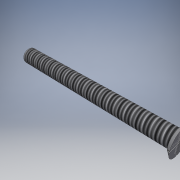
# Autodesk Inventor part: screws (for assembly)
Saved by Autodesk Inventor 2016 (Build 200138000, 138)
## iProperties
Created: 2017-10-23
Part Number: screws (for assembly)
Material: Generic
Document SubType Name: Modeling
Designer: student
Density: 1 g/cm^3
Appearance: Default
Author: student
Autodesk Inventor part; units mm, degrees
ref_plane "YZ Plane" through (0, 0, 0) normal (1, 0, 0) x (0, 1, 0)
ref_plane "XZ Plane" through (0, 0, 0) normal (0, 1, 0) x (-1, 0, 0)
ref_plane "XY Plane" through (0, 0, 0) normal (0, 0, 1) x (1, 0, 0)
sketch "Sketch1" plane through (0, 0, 0) normal (1, 0, 0) x (0, 1, 0)
  circle A0 centre (0, 0) radius 3.175
  dimension "d0" = 6.35
  constraints: 1 centre point, 1 coincident
  measures "d0" diameter of A0
extrude "Extrusion1" add sketch "Sketch1" against normal blind 63.5
sketch "Sketch2" plane through (0, 0, 0) normal (1, 0, 0) x (0, 0, -1)
  circle A0 centre (0, 0) radius 3.175 projected
  circle A1 centre (0, 0) radius 5.08
  dimension "d3" = 10.16
  constraints: 1 centre point, 1 coincident
  measures "d3" diameter of A1
extrude "Extrusion2" add sketch "Sketch2" along normal blind 1.27 contours A0 | A1
chamfer "Chamfer1" distance 1.27 angle 45 1 edges at (0, 0, 5.08)
sketch "Sketch3" plane through (1.27, 0, 0) normal (1, 0, 0) x (0, 0, -1)
  line L0 (-0.254, -5.08) -> (0.254, -5.08)
  line L1 (0.254, -5.08) -> (0.254, 5.08)
  line L2 (0.254, 5.08) -> (-0.254, 5.08)
  line L3 (-0.254, 5.08) -> (-0.254, -5.08)
  line L4 (-0.254, -5.08) -> (0.254, 5.08) construction
  line L5 (0.254, -5.08) -> (-0.254, 5.08) construction
  line L6 (-5.08, -0.254) -> (5.08, -0.254)
  line L7 (5.08, -0.254) -> (5.08, 0.254)
  line L8 (5.08, 0.254) -> (-5.08, 0.254)
  line L9 (-5.08, 0.254) -> (-5.08, -0.254)
  line L10 (-5.08, -0.254) -> (5.08, 0.254) construction
  line L11 (5.08, -0.254) -> (-5.08, 0.254) construction
  point P0 (0, 0)
  dimension "d9" = 0.508
  dimension "d10" = 10.16
  dimension "d11" = 10.16
  dimension "d12" = 0.508
  constraints: 24 end point, 4 midpoint, 4 parallel, 2 horizontal, 2 perpendicular
  measures "d9" distance of L1.end L2.end
  measures "d10" distance of L0.end L1.end
  measures "d11" distance of L7.end L8.end
  measures "d12" distance of L6.end L7.end
extrude "Extrusion3" cut sketch "Sketch3" against normal blind 0.508
thread "Thread1" size "1/4-20 UNC" class "2A" standard "ANSI Unified Screw Threads" full length
thread "Thread2" size "1-8 UNC" class "2A" standard "ANSI Unified Screw Threads" full length
body "Solid1"
